Autodesk Inventor part; units mm, degrees
(part 2 of 2)
equation "\"d320\" = 14.05"
equation "\"d323\" = 14.05"
equation "\"d326\" = 14.05"
equation "\"d329\" = 14.05"
equation "\"keym\" = 2"
equation "\"d476\" = 17.05"
equation "\"d477\" = 6.05"
equation "\"d480\" = 17.05"
equation "\"d481\" = 6.05"
equation "\"d484\" = 17.05"
equation "\"d485\" = 6.05"
equation "\"d488\" = 17.05"
equation "\"d489\" = 6.05"
equation "\"d492\" = 17.05"
equation "\"d493\" = 6.05"
equation "\"d496\" = 17.05"
equation "\"d497\" = 6.05"
equation "\"d500\" = 17.05"
equation "\"d501\" = 6.05"
equation "\"d506\" = 6.05"
equation "\"d507\" = 17.05"
body "Solid2"
body "Solid4"
